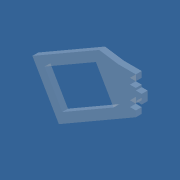
# Autodesk Inventor part: acrylic kinect bracket
Saved by Autodesk Inventor 2012 (Build 160160000, 160)
## iProperties
Created: 2012-10-30
Part Number: acrylic kinect bracket
Material: Default
Document SubType Name: Modeling
Designer: Ed
Density: 1 g/cm^3
Author: Ed
Autodesk Inventor part; units mm, degrees
note: some values were not read from the file. Chosen so that the rebuilt part matches the saved one: sketch regions of "Extrusion1".
ref_plane "YZ Plane" through (0, 0, 0) normal (1, 0, 0) x (0, 1, 0)
ref_plane "XZ Plane" through (0, 0, 0) normal (0, 1, 0) x (-1, 0, 0)
ref_plane "XY Plane" through (0, 0, 0) normal (0, 0, 1) x (1, 0, 0)
sketch "Sketch1" plane through (0, 0, 0) normal (0, 0, 1) x (1, 0, 0)
  line L0 (-98.4355, -21.9546) -> (-43.0099, 10.0454)
  line L1 (-43.0099, 10.0454) -> (-24.0099, -22.8636)
  line L2 (-24.0099, -22.8636) -> (-79.4355, -54.8636)
  line L3 (-79.4355, -54.8636) -> (-98.4355, -21.9546)
  line L4 (-6.35, -7.3) -> (0, -7.3)
  line L5 (0, -7.3) -> (0, -13.65)
  line L6 (0, -13.65) -> (-6.35, -13.65)
  line L7 (-6.35, -13.65) -> (-6.35, -7.3)
  line L8 (6.35, -4.953) -> (0, -4.953)
  line L9 (0, -4.953) -> (0, 4.953)
  line L10 (0, 4.953) -> (6.35, 4.953)
  line L11 (6.35, 4.953) -> (6.35, -4.953)
  line L12 (-6.35, 13.65) -> (0, 13.65)
  line L13 (0, 13.65) -> (0, 7.3)
  line L14 (0, 7.3) -> (-6.35, 7.3)
  line L15 (-6.35, 7.3) -> (-6.35, 13.65)
  line L16 (0, -20) -> (-19.05, -20)
  line L17 (-19.05, -20) -> (-19.05, 20)
  line L18 (-19.05, 20) -> (0, 20)
  line L19 (0, 20) -> (0, -20)
  line L20 (-10.9985, -26.35) -> (-39.5235, 23.0567)
  line L21 (-39.5235, 23.0567) -> (-111.4469, -18.4683)
  line L22 (-111.4469, -18.4683) -> (-82.9219, -67.875)
  line L23 (-82.9219, -67.875) -> (-10.9985, -26.35)
  line L24 (-10.9985, -26.35) -> (0, -20)
  line L25 (-19.05, 20) -> (-39.5235, 23.0567)
  point P0 (0, 0)
  point P1 (0, 0)
  dimension "d0" = 6.35
  dimension "d2" = 9.906
  dimension "d3" = 40
  dimension "d4" = 6.35
  dimension "d5" = 6.35
  dimension "d6" = 6.35
  dimension "d7" = 38
  dimension "d8" = 64
  dimension "d9" = 9.525
  dimension "d10" = 30
  dimension "d11" = 19.05
  dimension "d12" = 12.7
  constraints: 52 end point, 12 parallel, 6 perpendicular, 4 collinear, 4 horizontal, 3 equal length, 2 midpoint, 1 coincident, 3 other
  measures "d0" distance of L12.end L13.end
  measures "d2" distance of L10.end L8.start
  measures "d3" distance of L18.end L16.start
  measures "d4" distance of L9.end L10.end
  measures "d5" distance between parallel lines of L18 L12
  measures "d6" distance between parallel lines of L16 L6
  measures "d7" distance of L2.end L0.start
  measures "d8" distance of L0.start L0.end
  measures "d9" distance between parallel lines of L2 L23
  measures "d10" angle of L16 L24
  measures "d11" distance of L17.end L18.end
  measures "d12" distance of L20.start L16.start
extrude "Extrusion1" add sketch "Sketch1" along normal blind 6.35 contours L7 L6 L19 L16 L20 L17 L18 L12 L15 L14 L9 L4 | L9 L10 L11 L8 | L24 L20 L16 | L20 L23 L22 L21 L17 L16 | L16 L17 L20 | L20 L25 L17
body "Solid1"
